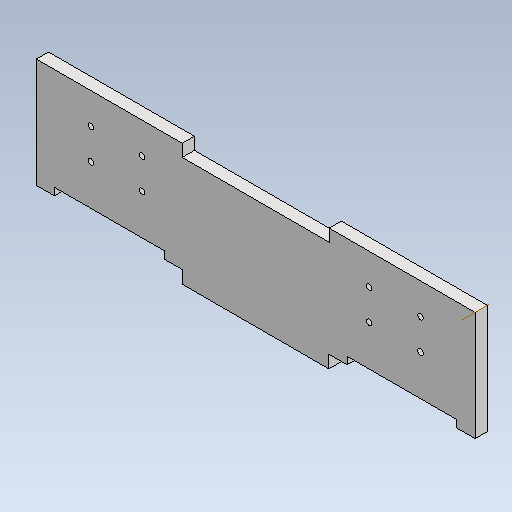
# Autodesk Inventor part: upper-front-plate-support
Saved by Autodesk Inventor 2025 (Build 290162000, 162)
## iProperties
Created: 2025-08-21
Part Number: upper-front-plate-support
Material: Glass
Document SubType Name: Modeling
Designer: HP
Density: 2.18 g/cm^3
Appearance: Default
Author: HP
Autodesk Inventor part; units mm, degrees
ref_plane "YZ Plane" through (0, 0, 0) normal (1, 0, 0) x (0, 1, 0)
ref_plane "XZ Plane" through (0, 0, 0) normal (0, 1, 0) x (-1, 0, 0)
ref_plane "XY Plane" through (0, 0, 0) normal (0, 0, 1) x (1, 0, 0)
sketch "Sketch1" plane through (0, 0, 0) normal (0, 0, 1) x (1, 0, 0)
  line L0 (-89.9, -25) -> (89.9, -25)
  line L1 (89.9, -25) -> (89.9, 25)
  line L2 (89.9, 25) -> (-89.9, 25)
  line L3 (-89.9, 25) -> (-89.9, -25)
  line L4 (-89.9, -25) -> (89.9, 25) construction
  line L5 (89.9, -25) -> (-89.9, 25) construction
  line L6 (46.5, 12.25) -> (67.5, 12.25) construction
  line L7 (67.5, 12.25) -> (67.5, -0.25) construction
  line L8 (67.5, -0.25) -> (46.5, -0.25) construction
  line L9 (46.5, -0.25) -> (46.5, 12.25) construction
  line L10 (46.5, 12.25) -> (67.5, -0.25) construction
  line L11 (67.5, 12.25) -> (46.5, -0.25) construction
  circle A0 centre (46.5, 12.25) radius 1.15
  circle A1 centre (67.5, 12.25) radius 1.15
  circle A2 centre (67.5, -0.25) radius 1.15
  circle A3 centre (46.5, -0.25) radius 1.15
  line L12 (-30.1, 25) -> (30.1, 25)
  line L13 (30.1, 25) -> (30.1, 20)
  line L14 (30.1, 20) -> (-30.1, 20)
  line L15 (-30.1, 20) -> (-30.1, 25)
  line L16 (-30.1, 25) -> (30.1, 20) construction
  line L17 (30.1, 25) -> (-30.1, 20) construction
  line L18 (-89.9, -19.8) -> (-30, -19.8)
  line L19 (-30, -19.8) -> (-30, -25)
  line L20 (-30, -25) -> (-89.9, -25)
  line L21 (-89.9, -25) -> (-89.9, -19.8)
  line L22 (-89.9, -19.8) -> (-30, -25) construction
  line L23 (-30, -19.8) -> (-89.9, -25) construction
  line L24 (19.7182, -25) -> (70.1, -25)
  line L25 (0, 0) -> (0, -25) construction
  line L26 (30, -25) -> (89.9, -25)
  line L27 (89.9, -25) -> (89.9, -19.8)
  line L28 (89.9, -19.8) -> (30, -19.8)
  line L29 (30, -19.8) -> (30, -25)
  line L30 (30, -25) -> (89.9, -19.8) construction
  line L31 (89.9, -25) -> (30, -19.8) construction
  line L32 (37.45, -16.8) -> (82.45, -16.8)
  line L33 (82.45, -16.8) -> (82.45, -19.8)
  line L34 (82.45, -19.8) -> (37.45, -19.8)
  line L35 (37.45, -19.8) -> (37.45, -16.8)
  line L36 (37.45, -16.8) -> (82.45, -19.8) construction
  line L37 (82.45, -16.8) -> (37.45, -19.8) construction
  point P0 (57, 6)
  point P1 (0, 22.5)
  point P2 (-59.95, -22.4)
  point P3 (30.1, 25)
  point P4 (-30.1, 25)
  point P5 (59.95, -22.4)
  point P6 (30, -25)
  point P7 (59.95, -18.3)
  point P8 (37.45, -19.8)
  dimension "d0" = 179.8
  dimension "d1" = 50
  dimension "d2" = 12.5
  dimension "d3" = 21
  dimension "d4" = 2.3
  dimension "d5" = 2.3
  dimension "d6" = 2.3
  dimension "d7" = 2.3
  dimension "d8" = 57
  dimension "d9" = 6
  dimension "d10" = 5
  dimension "d11" = 60.2
  dimension "d12" = 5.2
  dimension "d21" = 5.2
  dimension "d24" = 60
  dimension "d25" = 45
  dimension "d26" = 3
  constraints: 76 end point, 13 midpoint, 12 parallel, 7 collinear, 7 horizontal, 6 perpendicular, 4 centre point, 4 coincident, 2 vertical alignment, 1 other
  measures "d0" distance between parallel lines of L1 L3
  measures "d1" distance between parallel lines of L0 L2
  measures "d2" distance between parallel lines of L8 L6
  measures "d3" distance between parallel lines of L7 L9
  measures "d4" diameter of A0
  measures "d5" diameter of A1
  measures "d6" diameter of A2
  measures "d7" diameter of A3
  measures "d8" horizontal distance of point (57, 6) L25.start
  measures "d9" vertical distance of L25.start point (57, 6)
  measures "d10" distance between parallel lines of L14 L12
  measures "d11" distance between parallel lines of L15 L13
  measures "d12" distance between parallel lines of L20 L18
  measures "d21" distance between parallel lines of L26 L28
  measures "d24" distance between parallel lines of L29 L19
  measures "d25" distance of L33.end L34.end
  measures "d26" distance between parallel lines of L34 L32
extrude "Extrusion1" add sketch "Sketch1" along normal blind 5 contours L19 L18 L3 L2 L15 L14 L13 L1 L28 L33 L32 L35 L29 L0 | L35 L32 L33 L28 | A0 | A1 | A2 | A3
extrude "Extrusion2" cut sketch "Sketch1" along normal through all contours L35 L32 L33 L28 | A0 | A1 | A2 | A3
mirror "Mirror1" about plane through (0, 0, 0) normal (1, 0, 0) of "Extrusion2"
equation "\"d5\" = d4"
equation "\"d6\" = d5"
equation "\"d7\" = d4"
body "Solid1"
